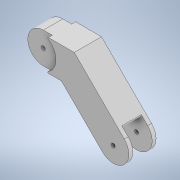
# Autodesk Inventor part: Arm2
Saved by Autodesk Inventor 2021 (Build 250183000, 183)
## iProperties
Created: 2024-09-30
Part Number: Arm2
Material: Generic
Document SubType Name: Modeling
Designer: Swoby
Density: 1 g/cm^3
Appearance: Default
Author: Swoby
Autodesk Inventor part; units mm, degrees
ref_plane "YZ Plane" through (0, 0, 0) normal (1, 0, 0) x (0, 1, 0)
ref_plane "XZ Plane" through (0, 0, 0) normal (0, 1, 0) x (-1, 0, 0)
ref_plane "XY Plane" through (0, 0, 0) normal (0, 0, 1) x (1, 0, 0)
sketch "Sketch1" plane through (0, 0, 0) normal (0, 0, 1) x (1, 0, 0)
  arc A0 (0, 40) -> (0, -40) centre (0, 0) ccw
  arc A1 (161.7157, -145.2843) -> (218.2843, -88.7157) centre (190, -117) ccw
  line L0 (0, 40) -> (89.5685, 40)
  line L1 (89.5685, 40) -> (218.2843, -88.7157)
  line L2 (0, -40) -> (56.4315, -40)
  line L3 (56.4315, -40) -> (161.7157, -145.2843)
  arc A2 (0, -40) -> (0, 40) centre (0, 0) ccw construction
  arc A3 (218.2843, -88.7157) -> (161.7157, -145.2843) centre (190, -117) ccw construction
  circle A4 centre (0, 0) radius 5
  circle A5 centre (190, -117) radius 5
  line L4 (0, -40) -> (161.7157, -40)
  line L5 (93.4315, -77) -> (190, -77)
  dimension "d0" = 80
  dimension "d1" = 80
  dimension "d2" = 190
  dimension "d3" = 117
  dimension "d4" = 135
  dimension "d9" = 10
  dimension "d10" = 10
  constraints: 12 end point, 9 point on circle, 7 tangent, 6 centre point, 3 coincident, 3 parallel, 2 point on line, 1 horizontal
  measures "d0" diameter of A0
  measures "d1" diameter of A1
  measures "d2" horizontal distance of A1.centre point (0, 0)
  measures "d3" vertical distance of A1.centre point (0, 0)
  measures "d4" angle of L1 L0
  measures "d9" diameter of A4
  measures "d10" diameter of A5
extrude "Extrusion1" add sketch "Sketch1" along normal mid plane 70
sketch "Sketch2" plane through (0, 0, 0) normal (0, 0, 1) x (1, 0, 0)
  arc A0 (0, 40) -> (0, -40) centre (0, 0) ccw projected
  line L0 (0, -40) -> (56.4315, -40) projected
  line L1 (56.4315, -40) -> (161.7157, -145.2843) projected
  arc A1 (161.7157, -145.2843) -> (218.2843, -88.7157) centre (190, -117) ccw projected
  line L2 (218.2843, -88.7157) -> (89.5685, 40) projected
  line L3 (89.5685, 40) -> (0, 40) projected
  circle A2 centre (0, 0) radius 42.5
  circle A3 centre (190, -117) radius 42.5
  point P0 (208.1292, -78.5607)
  point P1 (151.5607, -135.1292)
  dimension "d7" = 85
  dimension "d8" = 85
  constraints: 2 centre point, 2 coincident
  measures "d7" diameter of A2
  measures "d8" diameter of A3
extrude "Extrusion2" cut sketch "Sketch2" along normal mid plane 50 contours L2 A1 L1 A3 picked at (179.9827, -106.9827)
sketch "Sketch3" plane through (0, 0, 35) normal (0, 0, 1) x (1, 0, 0)
  arc A0 (0, 40) -> (0, -40) centre (0, 0) ccw projected
  line L0 (0, -40) -> (56.4315, -40) projected
  line L1 (56.4315, -40) -> (161.7157, -145.2843) projected
  arc A1 (161.7157, -145.2843) -> (218.2843, -88.7157) centre (190, -117) ccw projected
  line L2 (218.2843, -88.7157) -> (89.5685, 40) projected
  line L3 (89.5685, 40) -> (0, 40) projected
  circle A2 centre (0, 0) radius 5 projected
  circle A3 centre (190, -117) radius 5 projected
  circle A4 centre (0, 0) radius 42.5
  dimension "d13" = 85
  constraints: 1 centre point, 1 coincident
  measures "d13" diameter of A4
extrude "Extrusion3" cut sketch "Sketch3" against normal blind 10 contours L3 A4 L0 A0 | A0 L0 A4 L3 | A2
mirror "Mirror1" about plane through (0, 0, 0) normal (0, 0, 1) of "Extrusion3"
fillet "Fillet1" radius 2 6 edges at (14.3614, 40, -30) (14.3614, 40, 30) (14.3614, -40, 30) (14.3614, -40, -30) (151.5607, -135.1292, 0) (208.1292, -78.5607, 0)
body "Solid1"
